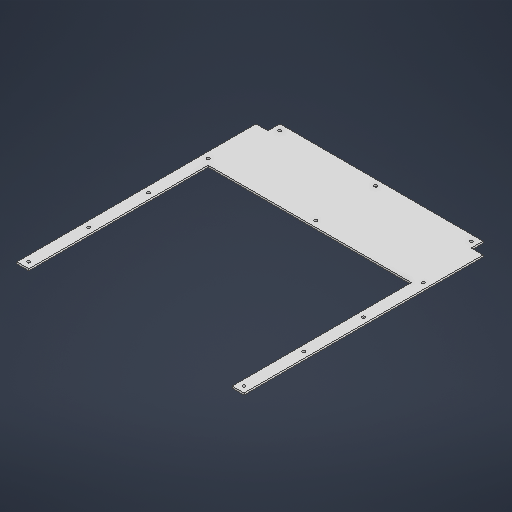
# Autodesk Inventor part: CaraMedia
Saved by Autodesk Inventor 2026.2 (Build 302298010, 298A)
## iProperties
Created: 2026-04-15
Part Number: CaraMedia
Material: Generic
Document SubType Name: Modeling
Designer: grego
Density: 1 g/cm^3
Appearance: Default
Author: grego
Autodesk Inventor part; units mm, degrees
ref_plane "YZ Plane" through (0, 0, 0) normal (1, 0, 0) x (0, 1, 0)
ref_plane "XZ Plane" through (0, 0, 0) normal (0, 1, 0) x (-1, 0, 0)
ref_plane "XY Plane" through (0, 0, 0) normal (0, 0, 1) x (1, 0, 0)
sketch "Sketch1" plane through (0, 0, 0) normal (0, 1, 0) x (-1, 0, 0)
  line L0 (190, 210) -> (190, -210)
  line L1 (190, -210) -> (-190, -210)
  line L2 (-190, -210) -> (-190, 210)
  line L3 (-170, -190) -> (170, -190)
  line L4 (170, -190) -> (170, 190)
  line L5 (-170, 190) -> (-170, -190)
  line L6 (-180, -200) -> (180, -200)
  line L7 (180, -200) -> (180, 200)
  line L8 (-180, 200) -> (-180, -200)
  line L9 (190, -210) -> (190, -90)
  line L10 (190, -90) -> (-190, -90)
  line L11 (170, 190) -> (170, 210)
  line L12 (180, 200) -> (180, 210)
  line L13 (-170, 190) -> (-170, 210)
  line L14 (-180, 200) -> (-180, 210)
  line L15 (-190, 210) -> (-170, 210)
  line L16 (170, 210) -> (190, 210)
  line L17 (190, -90) -> (190, -100)
  line L18 (190, -100) -> (-190, -100)
  line L19 (190, -100) -> (190, -110)
  line L20 (190, -110) -> (-190, -110)
  circle A0 centre (180, 200) radius 2.5
  circle A1 centre (-180, 200) radius 2.5
  circle A2 centre (180, -100) radius 2.5
  circle A3 centre (-180, -100) radius 2.5
  circle A4 centre (0, -100) radius 2.5
  circle A5 centre (180, 100) radius 2.5
  circle A6 centre (180, 0) radius 2.5
  line L21 (0, 0) -> (0, 25.5231)
  circle A7 centre (-180, 100) radius 2.5
  circle A8 centre (-180, 0) radius 2.5
  circle A9 centre (0, -200) radius 2.5
  circle A10 centre (160, -200) radius 2.5
  circle A11 centre (-160, -200) radius 2.5
  point P0 (170, -90)
  point P1 (-170, -90)
  dimension "d0" = 380
  dimension "d1" = 420
  dimension "d2" = 20
  dimension "d3" = 10
  dimension "d4" = 120
  dimension "d5" = 10
  dimension "d6" = 10
  dimension "d7" = 5
  dimension "d8" = 5
  dimension "d9" = 5
  dimension "d10" = 5
  dimension "d11" = 5
  dimension "d12" = 5
  dimension "d13" = 5
  dimension "d14" = 5
  dimension "d15" = 5
  dimension "d16" = 5
  constraints: 44 end point, 13 perpendicular, 13 point on line, 12 centre point, 5 midpoint, 5 parallel, 2 coincident, 2 horizontal, 2 symmetric about line, 1 vertical, 4 other
  measures "d0" distance of L0.end L1.end
  measures "d1" distance of L0.start L0.end
  measures "d2" distance between parallel lines of L1 L3
  measures "d3" distance between parallel lines of L1 L6
  measures "d4" distance of L0.end L9.end
  measures "d5" distance of L9.end L17.end
  measures "d6" distance of L17.end L19.end
  measures "d7" diameter of A0
  measures "d8" diameter of A1
  measures "d9" diameter of A2
  measures "d10" diameter of A3
  measures "d11" diameter of A4
  measures "d12" diameter of A5
  measures "d13" diameter of A6
  measures "d14" diameter of A9
  measures "d15" diameter of A10
  measures "d16" diameter of A11
extrude "Extrusion1" add sketch "Sketch1" along normal blind 3 contours L0 L10 L7 A6 A5 A0 L12 L16 | L0 L18 A2 L7 L10 | L12 A0 L7 A5 A6 L10 L4 L11 L16 | L0 L20 L7 A2 L18 | L7 A2 L18 L4 L10 | L0 L1 L2 L20 L8 L6 A11 A9 A10 L7 | L4 L18 A4 L5 L10 | L20 L4 L18 A2 L7 | L7 L6 A10 A9 A11 L8 L20 L5 L3 L4 | L4 L20 L5 L18 A4 | L10 L8 A8 A7 A1 L14 L15 L13 L5 | L5 L18 A3 L8 L10 | L4 L3 L5 L20 | L5 L20 L8 A3 L18 | L10 L2 L15 L14 A1 L8 A7 A8 | L8 A3 L18 L2 L10 | L2 L18 A3 L8 L20
sketch "Sketch2" plane through (0, 3, 0) normal (0, 1, 0) x (1, 0, 0)
  line L0 (170, 90) -> (170, -210) projected
  line L1 (170, -210) -> (190, -210) projected
  line L2 (190, -210) -> (190, 210) projected
  line L3 (190, 210) -> (-190, 210) projected
  line L4 (-190, 210) -> (-190, -210) projected
  line L5 (-190, -210) -> (-170, -210) projected
  line L6 (-170, -210) -> (-170, 90) projected
  line L7 (-170, 90) -> (170, 90) projected
  circle A0 centre (-180, -200) radius 2.5 projected
  circle A1 centre (-180, -100) radius 2.5 projected
  circle A2 centre (-180, 0) radius 2.5 projected
  circle A3 centre (180, 100) radius 2.5 projected
  circle A4 centre (180, 0) radius 2.5 projected
  circle A5 centre (180, -100) radius 2.5 projected
  circle A6 centre (180, -200) radius 2.5 projected
  circle A7 centre (0, 100) radius 2.5 projected
  circle A8 centre (160, 200) radius 2.5 projected
  circle A9 centre (0, 200) radius 2.5 projected
  circle A10 centre (-160, 200) radius 2.5 projected
  circle A11 centre (-180, 100) radius 2.5 projected
  line L8 (-190, 210) -> (-170, 210)
  line L9 (-170, 210) -> (-170, 190)
  line L10 (-170, 190) -> (-190, 190)
  line L11 (-190, 190) -> (-190, 210)
  line L12 (190, 210) -> (170, 210)
  line L13 (170, 210) -> (170, 190)
  line L14 (170, 190) -> (190, 190)
  line L15 (190, 190) -> (190, 210)
  point P0 (0, 0)
  dimension "d19" = 20
  dimension "d20" = 20
  dimension "d21" = 20
  dimension "d22" = 20
  constraints: 16 end point, 4 parallel, 2 horizontal, 2 perpendicular
  measures "d19" distance of L9.end L10.end
  measures "d20" distance of L8.end L9.end
  measures "d21" distance of L14.end L13.end
  measures "d22" distance of L13.end L12.end
extrude "Extrusion2" cut sketch "Sketch2" against normal blind 3 contours L14 L13 L3 L2 | L4 L3 L9 L10
body "Solid1"
